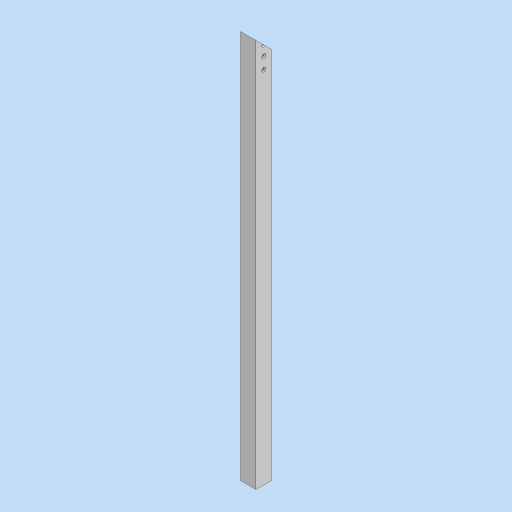
# Autodesk Inventor part: STRU_005_BilletPole_25in_Angled
Saved by Autodesk Inventor 2024.3 (Build 283343000, 343)
## iProperties
Created: 2024-07-23
Part Number: STRU_005_BilletPole_25in_Angled
Material: Generic
Document SubType Name: Modeling
Designer: bryan
Density: 1 g/cm^3
Appearance: Default
Author: bryan
Autodesk Inventor part; units mm, degrees
ref_plane "YZ Plane" through (0, 0, 0) normal (1, 0, 0) x (0, 1, 0)
ref_plane "XZ Plane" through (0, 0, 0) normal (0, 1, 0) x (-1, 0, 0)
ref_plane "XY Plane" through (0, 0, 0) normal (0, 0, 1) x (1, 0, 0)
sketch "Sketch1" plane through (0, 0, 0) normal (0, 1, 0) x (-1, 0, 0)
  line L0 (-12.7, -12.7) -> (12.7, -12.7)
  line L1 (12.7, -12.7) -> (12.7, 12.7)
  line L2 (12.7, 12.7) -> (-12.7, 12.7)
  line L3 (-12.7, 12.7) -> (-12.7, -12.7)
  line L4 (-12.7, -12.7) -> (12.7, 12.7) construction
  line L5 (12.7, -12.7) -> (-12.7, 12.7) construction
  line L6 (9.525, 9.525) -> (9.525, -9.525)
  line L7 (9.525, -9.525) -> (-9.525, -9.525)
  line L8 (-9.525, -9.525) -> (-9.525, 9.525)
  line L9 (-9.525, 9.525) -> (9.525, 9.525)
  point P0 (0, 0)
  dimension "d0" = 25.4
  dimension "d1" = 25.4
  dimension "d2" = 3.175
  constraints: 20 end point, 4 parallel, 2 midpoint, 2 perpendicular, 1 horizontal, 3 other
  measures "d0" distance of L2.end L1.end
  measures "d1" distance of L1.end L0.end
  measures "d2" distance between parallel lines of L1 L6
extrude "Extrusion1" add sketch "Sketch1" along normal blind 635
sketch "Sketch2" plane through (12.7, 0, 12.7) normal (1, 0, 0) x (0, 0, -1)
  line L0 (25.4, 635) -> (0, 635) projected
  line L1 (0, 635) -> (25.4, 609.6)
  line L2 (25.4, 0) -> (25.4, 635) projected
  circle A0 centre (12.7, 622.3) radius 3.2512
  circle A1 centre (12.7, 606.425) radius 3.2512
  circle A2 centre (12.7, 587.375) radius 3.2512
  point P0 (12.7, 0)
  point P1 (10.4011, 624.5989)
  point P2 (14.9989, 620.0011)
  dimension "d5" = 25.4
  dimension "d6" = 6.5024
  dimension "d7" = 28.575
  dimension "d8" = 19.05
  constraints: 3 centre point, 2 end point, 2 equal radius, 1 midpoint, 1 point on line
  measures "d5" distance of L1.end L0.start
  measures "d6" diameter of A0
  measures "d7" distance from line of L0 A1.centre
  measures "d8" distance of A1.centre A2.centre
extrude "Extrusion2" cut sketch "Sketch2" against normal through all
body "Solid1"
